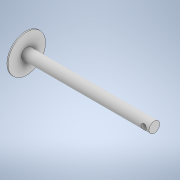
# Autodesk Inventor part: Intake Basic Piston - Inner
Saved by Autodesk Inventor 2020 (Build 240168000, 168)
## iProperties
Created: 2020-02-04
Part Number: Intake Basic Piston - Inner
Material: Generic
Document SubType Name: Modeling
Designer: aidan
Density: 1 g/cm^3
Appearance: Default
Author: aidan
Autodesk Inventor part; units mm, degrees
ref_plane "YZ Plane" through (0, 0, 0) normal (1, 0, 0) x (0, 1, 0)
ref_plane "XZ Plane" through (0, 0, 0) normal (0, 1, 0) x (-1, 0, 0)
ref_plane "XY Plane" through (0, 0, 0) normal (0, 0, 1) x (1, 0, 0)
sketch "Sketch1" plane through (0, 0, 0) normal (1, 0, 0) x (0, 1, 0)
  circle A0 centre (0, 0) radius 22.225
  dimension "d0" = 44.45
  constraints: 1 centre point, 1 coincident
  measures "d0" diameter of A0
extrude "Extrusion1" add sketch "Sketch1" along normal blind 1.27
sketch "Sketch2" plane through (1.27, 0, 0) normal (1, 0, 0) x (0, 0, -1)
  circle A0 centre (0, 0) radius 6.35
  dimension "d3" = 12.7
  constraints: 1 centre point, 1 coincident
  measures "d3" diameter of A0
extrude "Extrusion2" add sketch "Sketch2" along normal blind 151.13
sketch "Sketch3" plane through (152.4, 0, 0) normal (1, 0, 0) x (0, 0, -1)
  circle A0 centre (0, 0) radius 6.35 projected
  circle A1 centre (0, 0) radius 6.35 projected
  point P0 (-6.35, 0)
  point P1 (6.35, 0)
  constraints: 2 point on circle
ref_plane "Work Plane3" through (152.4, 0, 0) normal (0, 0, -1) x (-1, 0, 0)
ref_plane "Work Plane1" through (152.4, 0, 6.35) normal (0, 0, 1) x (1, 0, 0)
ref_plane "Work Plane2" through (152.4, 0, -6.35) normal (0, 0, -1) x (-1, 0, 0)
sketch "Sketch4" plane through (152.4, 0, -6.35) normal (0, 0, -1) x (-1, 0, 0)
  circle A0 centre (6.35, 0) radius 3.175
  line L0 (0, 6.35) -> (0, -6.35) projected
  point P0 (152.4, 0)
  dimension "d6" = 6.35
  dimension "d7" = 6.35
  constraints: 1 centre point
  measures "d6" diameter of A0
  measures "d7" distance from line of L0 A0.centre
extrude "Extrusion3" cut sketch "Sketch4" against normal blind 12.7
body "Solid1"
